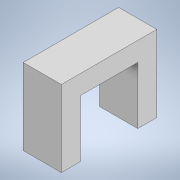
# Autodesk Inventor part: attach
Saved by Autodesk Inventor 2020 (Build 240168000, 168)
## iProperties
Created: 2021-07-09
Part Number: attach
Material: Generic
Document SubType Name: Modeling
Designer: pc
Density: 1 g/cm^3
Appearance: Default
Author: pc
Autodesk Inventor part; units mm, degrees
ref_plane "YZ Plane" through (0, 0, 0) normal (1, 0, 0) x (0, 1, 0)
ref_plane "XZ Plane" through (0, 0, 0) normal (0, 1, 0) x (-1, 0, 0)
ref_plane "XY Plane" through (0, 0, 0) normal (0, 0, 1) x (1, 0, 0)
sketch "Sketch1" plane through (0, 0, 0) normal (1, 0, 0) x (0, 1, 0)
  line L0 (-45.4409, 46.5335) -> (5.3591, 46.5335)
  line L1 (5.3591, 46.5335) -> (5.3591, -16.9665)
  line L2 (5.3591, -16.9665) -> (-45.4409, -16.9665)
  line L3 (-45.4409, 46.5335) -> (-45.4409, 33.8335)
  line L4 (-45.4409, 33.8335) -> (-7.3409, 33.8335)
  line L5 (-7.3409, 33.8335) -> (-7.3409, -4.2665)
  line L6 (-7.3409, -4.2665) -> (-45.4409, -4.2665)
  line L7 (-45.4409, -4.2665) -> (-45.4409, -16.9665)
  point P0 (0, 0)
  dimension "d0" = 63.5
  dimension "d1" = 50.8
  dimension "d2" = 50.8
  dimension "d3" = 12.7
  dimension "d4" = 38.1
  dimension "d5" = 38.1
  constraints: 16 end point, 3 perpendicular, 1 horizontal
  measures "d0" distance of L0.end L1.end
  measures "d1" distance of L0.start L0.end
  measures "d2" distance of L1.end L2.end
  measures "d3" distance of L0.start L3.end
  measures "d4" distance of L3.end L4.end
  measures "d5" distance of L4.end L5.end
extrude "Extrusion1" add sketch "Sketch1" along normal blind 25.4
body "Solid1"
